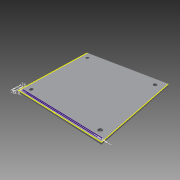
# Autodesk Inventor part: Enclosure2
Saved by Autodesk Inventor 2015 (Build 190159000, 159)
## iProperties
Created: 2014-08-04
Part Number: Enclosure2
Material: Generic
Document SubType Name: Modeling
Designer: Patrick Camilleri
Density: 1 g/cm^3
Appearance: Default
Author: Patrick Camilleri
Autodesk Inventor part; units mm, degrees
ref_plane "YZ Plane" through (0, 0, 0) normal (1, 0, 0) x (0, 1, 0)
ref_plane "XZ Plane" through (0, 0, 0) normal (0, 1, 0) x (-1, 0, 0)
ref_plane "XY Plane" through (0, 0, 0) normal (0, 0, 1) x (1, 0, 0)
sketch "Sketch1" plane through (0, 0, 0) normal (0, 1, 0) x (-1, 0, 0)
  line L0 (220, 120) -> (0, 120)
  line L1 (0, 120) -> (0, -120)
  line L2 (0, -120) -> (220, -120)
  line L3 (220, -120) -> (220, 120)
  point P0 (0, 0)
  dimension "d0" = 220
  dimension "d1" = 240
  constraints: 8 end point, 2 parallel, 1 horizontal, 1 perpendicular
  measures "d0" distance of L1.end L2.end
  measures "d1" distance of L0.end L1.end
extrude "Extrusion1" add sketch "Sketch1" along normal blind 6
sketch "Sketch2" plane through (0, 6, 0) normal (0, 1, 0) x (1, 0, 0)
  line L0 (-220, -120) -> (0, -120) projected
  line L1 (0, -120) -> (0, 120) projected
  point P0 (0, 0)
  point P1 (-20, -100)
  point P2 (-20, 100)
  point P3 (-200, -100)
  point P4 (-200, 100)
  dimension "d4" = 20
  dimension "d5" = 20
  dimension "d8" = 200
  dimension "d11" = 180
  constraints: 1 horizontal, 1 vertical, 3 other
  measures "d4" distance from line of L0 point (-20, -100)
  measures "d5" distance from line of L1 point (-20, -100)
  measures "d8" distance of point (-20, -100) point (-20, 100)
  measures "d11" distance of point (-20, -100) point (-200, -100)
hole "Hole1" at (-20, 6, 100) at (-20, 6, -100) at (-200, 6, 100) at (-200, 6, -100) direction (0, -1, 0) diameter 10 end through all
sketch "Sketch5" plane through (0, 6, 0) normal (0, 1, 0) x (1, 0, 0)
  line L0 (-8, -115) -> (-5, -115)
  line L1 (-5, -115) -> (-5, 115)
  line L2 (-5, 115) -> (-8, 115)
  line L3 (-8, 115) -> (-8, -115)
  line L4 (0, -120) -> (0, 120) projected
  line L5 (0, 120) -> (-220, 120) projected
  line L6 (-220, -120) -> (0, -120) projected
  point P0 (0, 0)
  dimension "d27" = 3
  dimension "d28" = 5
  dimension "d30" = 5
  dimension "d32" = 5
  constraints: 8 end point, 2 parallel, 1 horizontal, 1 perpendicular
  measures "d27" distance between parallel lines of L3 L1
  measures "d28" distance between parallel lines of L4 L1
  measures "d30" distance between parallel lines of L5 L2
  measures "d32" distance from line of L6 L0.start
equation "\"d32\" = d30"
body "Solid1"
